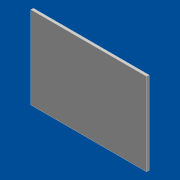
# Autodesk Inventor part: Base
Saved by Autodesk Inventor 2016 (Build 200138000, 138)
## iProperties
Created: 2017-05-14
Part Number: Base
Material: Generic
Document SubType Name: Modeling
Designer: Gian
Density: 1 g/cm^3
Appearance: Default
Author: Gian
Autodesk Inventor part; units mm, degrees
ref_plane "YZ Plane" through (0, 0, 0) normal (1, 0, 0) x (0, 1, 0)
ref_plane "XZ Plane" through (0, 0, 0) normal (0, 1, 0) x (-1, 0, 0)
ref_plane "XY Plane" through (0, 0, 0) normal (0, 0, 1) x (1, 0, 0)
sketch "Sketch1" plane through (0, 0, 0) normal (0, 1, 0) x (-1, 0, 0)
  line L0 (194.3776, -172.0551) -> (-505.6224, -172.0551)
  line L1 (-505.6224, -172.0551) -> (-505.6224, 327.9449)
  line L2 (-505.6224, 327.9449) -> (194.3776, 327.9449)
  line L3 (194.3776, 327.9449) -> (194.3776, -172.0551)
  line L4 (194.3776, -172.0551) -> (-505.6224, 327.9449) construction
  line L5 (-505.6224, -172.0551) -> (194.3776, 327.9449) construction
  point P0 (-155.6224, 77.9449)
  dimension "d2" = 700
  dimension "d3" = 500
  constraints: 12 end point, 2 midpoint, 2 parallel, 1 horizontal, 1 perpendicular
  measures "d2" distance of L0.start L0.end
  measures "d3" distance of L2.end L0.start
extrude "Extrusion1" add sketch "Sketch1" along normal blind 15
body "Solid1"
